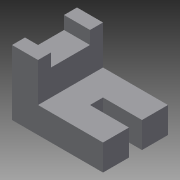
# Autodesk Inventor part: 7.1 Part 1
Saved by Autodesk Inventor 2015 (Build 190159000, 159)
## iProperties
Created: 2015-03-05
Part Number: 7.1 Part 1
Material: Generic
Document SubType Name: Modeling
Designer: PLTW-Stu-02
Density: 1 g/cm^3
Appearance: Default
Author: PLTW-Stu-02
Autodesk Inventor part; units mm, degrees
ref_plane "YZ Plane" through (0, 0, 0) normal (1, 0, 0) x (0, 1, 0)
ref_plane "XZ Plane" through (0, 0, 0) normal (0, 1, 0) x (-1, 0, 0)
ref_plane "XY Plane" through (0, 0, 0) normal (0, 0, 1) x (1, 0, 0)
sketch "Sketch1" plane through (0, 0, 0) normal (0, 0, 1) x (1, 0, 0)
  line L0 (13.4804, 26.8062) -> (26.1804, 26.8062)
  line L1 (57.9304, 7.7562) -> (57.9304, -4.9438)
  line L2 (57.9304, -4.9438) -> (13.4804, -4.9438)
  line L3 (13.4804, -4.9438) -> (13.4804, 26.8062)
  line L4 (26.1804, 26.8062) -> (26.1804, 7.7562)
  line L5 (26.1804, 7.7562) -> (57.9304, 7.7562)
  point P0 (0, 0)
  dimension "d0" = 44.45
  dimension "d3" = 19.05
  constraints: 12 end point, 2 parallel, 2 perpendicular, 1 horizontal, 1 vertical
  measures "d0" distance of L1.end L2.end
  measures "d3" distance of L0.end L4.end
extrude "Extrusion1" add sketch "Sketch1" along normal blind 31.75
sketch "Sketch3" plane through (57.9304, -4.9438, 0) normal (1, 0, 0) x (0, 0, -1)
  line L0 (-19.05, 12.7) -> (-12.7, 12.7)
  line L1 (-12.7, 12.7) -> (-12.7, 0)
  line L2 (-12.7, 0) -> (-19.05, 0)
  line L3 (-19.05, 0) -> (-19.05, 12.7)
  point P0 (0, 4.9438)
  constraints: 8 end point, 2 parallel, 1 horizontal, 1 perpendicular
extrude "Extrusion2" cut sketch "Sketch3" against normal blind 19.05
sketch "Sketch4" plane through (13.4804, 26.8062, 0) normal (0, 1, 0) x (1, 0, 0)
  line L0 (0, -25.4) -> (12.7, -25.4)
  line L1 (12.7, -25.4) -> (12.7, -6.35)
  line L2 (12.7, -6.35) -> (0, -6.35)
  line L3 (0, -6.35) -> (0, -25.4)
  point P0 (-13.4804, 0)
  dimension "d13" = 12.7
  dimension "d14" = 19.05
  constraints: 8 end point, 2 parallel, 1 horizontal, 1 perpendicular
  measures "d13" distance of L2.end L1.end
  measures "d14" distance of L1.end L0.end
extrude "Extrusion3" cut sketch "Sketch4" against normal blind 6.35
body "Solid1"
